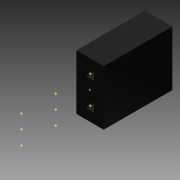
# Autodesk Inventor part: pwm connector 3 pin
Saved by Autodesk Inventor 2011 (Build 150239000, 239)
## iProperties
Created: 2010-02-11
Part Number: pwm connector 3 pin
Document SubType Name: Modeling
Designer: Kyle
Density: 1 g/cm^3
Author: Kyle
Autodesk Inventor part; units mm, degrees
ref_plane "YZ Plane" through (0, 0, 0) normal (1, 0, 0) x (0, 1, 0)
ref_plane "XZ Plane" through (0, 0, 0) normal (0, 1, 0) x (-1, 0, 0)
ref_plane "XY Plane" through (0, 0, 0) normal (0, 0, 1) x (1, 0, 0)
sketch "Sketch1" plane through (0, 0, 0) normal (0, 0, 1) x (1, 0, 0)
  line L0 (0.889, 1.651) -> (1.651, 1.651)
  line L1 (1.651, 1.651) -> (1.651, 0.889)
  line L2 (1.651, 0.889) -> (0.889, 0.889)
  line L3 (0.889, 0.889) -> (0.889, 1.651)
  line L4 (0.889, 4.191) -> (1.651, 4.191)
  line L5 (1.651, 4.191) -> (1.651, 3.429)
  line L6 (1.651, 3.429) -> (0.889, 3.429)
  line L7 (0.889, 3.429) -> (0.889, 4.191)
  line L8 (0, 5.08) -> (0, 0)
  line L9 (0, 0) -> (2.54, 0)
  line L10 (2.54, 0) -> (2.54, 5.08)
  line L11 (2.54, 5.08) -> (0, 5.08)
  point P0 (5.08, 24.13)
  constraints: 24 end point
extrude "Extrusion1" add sketch "Sketch1" along normal blind 6.35
ref_plane "Work Plane6" through (0, 0, 9.525) normal (0, 0, 1) x (1, 0, 0)
ref_plane "Work Plane7" through (0, 0, 12.7) normal (0, 0, 1) x (1, 0, 0)
ref_plane "Work Plane8" through (0, 0, 9.525) normal (0, 0, 1) x (1, 0, 0)
ref_plane "Work Plane9" through (0, 0, 12.7) normal (0, 0, 1) x (1, 0, 0)
ref_plane "Work Plane10" through (0, 0, 9.525) normal (0, 0, 1) x (1, 0, 0)
ref_plane "Work Plane11" through (0, 0, 12.7) normal (0, 0, 1) x (1, 0, 0)
body "Solid1"
